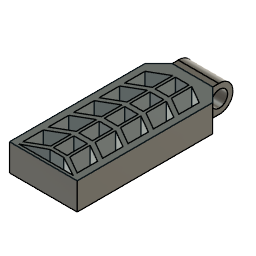
RocketAssembly_GridFin (Autodesk Fusion 360 design; units mm, degrees)
Autodesk Fusion 360 part; units mm, degrees
sketch "Sketch1" plane through (0, 0, 0) normal (0, 0, 1) x (1, 0, 0)
  line L0 (0, 0) -> (12.7, 0)
  line L1 (12.7, 0) -> (12.7, 25.4)
  line L2 (0, 25.4) -> (0, 0)
  line L3 (0, 25.4) -> (2.54, 27.94)
  line L4 (2.54, 27.94) -> (10.16, 27.94)
  line L5 (10.16, 27.94) -> (12.7, 25.4)
  dimension "d1" = 12.7
  dimension "d2" = 25.4
  constraint horizontal L0
  constraint vertical L1
  constraint vertical L2
  constraint coincident L0.start L2.end
  constraint perpendicular L2 L4
  measures "d1" distance of L0.start L0.end
  measures "d2" distance of L0.start L2.start
extrude "Extrude1" add sketch "Sketch1" along normal blind 5.08
sketch "Sketch2" plane through (12.7, 0, 0) normal (1, 0, 0) x (0, 1, 0)
  line L0 (0, 0) -> (25.4, 0)
  line L1 (25.4, 0) -> (25.4, 5.08)
  line L2 (25.4, 5.08) -> (0, 5.08)
  line L3 (0, 5.08) -> (0, 0)
  circle A0 centre (29.21, 2.54) radius 2.54
  circle A1 centre (29.21, 2.54) radius 1.524
  dimension "d5" = 3.048
  constraint concentric A0 A1
  measures "d5" diameter of A1
extrude "Extrude2" add sketch "Sketch2" along normal blind -2.54 and the other way blind 10.16 contours A0
fillet "Fillet1" radius 10.16 1 edges at (6.35, 27.94, 0.3403)
fillet "Fillet2" radius 10.16 1 edges at (6.35, 27.94, 4.7397)
sketch "Sketch3" plane through (0, 0, 5.08) normal (0, 0, 1) x (-1, 0, 0)
  line L0 (0, -25.4) -> (0, 0)
  line L1 (0, 0) -> (-12.7, 0)
  line L2 (-12.7, 0) -> (-12.7, -25.4)
  line L3 (-12.7, -25.4) -> (-10.16, -27.94)
  line L4 (-10.16, -27.94) -> (-2.54, -27.94)
  line L5 (-2.54, -27.94) -> (0, -25.4)
sketch "Sketch4" plane through (0, 0, 0) normal (0, 0, -1) x (1, 0, 0)
  line L0 (0, 0) -> (0, -25.4)
  line L1 (0, -25.4) -> (2.54, -27.94)
  line L2 (2.54, -27.94) -> (10.16, -27.94)
  line L3 (10.16, -27.94) -> (12.7, -25.4)
  line L4 (12.7, -25.4) -> (12.7, 0)
  line L5 (12.7, 0) -> (0, 0)
  line L6 (1.27, -1.27) -> (1.27, -5.08)
  line L7 (1.27, -5.08) -> (4.5696, -6.985)
  line L8 (1.27, -1.27) -> (4.5696, -3.175)
  line L9 (4.5696, -3.175) -> (4.5696, -6.985)
  line L10 (11.43, -1.27) -> (11.43, -5.08)
  line L11 (11.43, -5.08) -> (8.1304, -6.985)
  line L12 (8.1304, -6.985) -> (8.1304, -3.175)
  line L13 (8.1304, -3.175) -> (11.43, -1.27)
  line L14 (1.27, -9.8425) -> (4.5696, -11.7475)
  line L15 (1.27, -6.0325) -> (1.27, -9.8425)
  line L16 (1.27, -6.0325) -> (4.5696, -7.9375)
  line L17 (4.5696, -7.9375) -> (4.5696, -11.7475)
  line L18 (8.1304, -11.7475) -> (8.1304, -7.9375)
  line L19 (8.1304, -7.9375) -> (11.43, -6.0325)
  line L20 (11.43, -6.0325) -> (11.43, -9.8425)
  line L21 (11.43, -9.8425) -> (8.1304, -11.7475)
  line L22 (1.27, -14.605) -> (4.5696, -16.51)
  line L23 (1.27, -10.795) -> (1.27, -14.605)
  line L24 (1.27, -10.795) -> (4.5696, -12.7)
  line L25 (4.5696, -12.7) -> (4.5696, -16.51)
  line L26 (8.1304, -16.51) -> (8.1304, -12.7)
  line L27 (8.1304, -12.7) -> (11.43, -10.795)
  line L28 (11.43, -10.795) -> (11.43, -14.605)
  line L29 (11.43, -14.605) -> (8.1304, -16.51)
  line L30 (1.27, -19.3675) -> (4.5696, -21.2725)
  line L31 (1.27, -15.5575) -> (1.27, -19.3675)
  line L32 (1.27, -15.5575) -> (4.5696, -17.4625)
  line L33 (4.5696, -17.4625) -> (4.5696, -21.2725)
  line L34 (8.1304, -21.2725) -> (8.1304, -17.4625)
  line L35 (8.1304, -17.4625) -> (11.43, -15.5575)
  line L36 (11.43, -15.5575) -> (11.43, -19.3675)
  line L37 (11.43, -19.3675) -> (8.1304, -21.2725)
  line L38 (1.27, -24.13) -> (4.5696, -26.035)
  line L39 (1.27, -20.32) -> (1.27, -24.13)
  line L40 (1.27, -20.32) -> (4.5696, -22.225)
  line L41 (4.5696, -22.225) -> (4.5696, -26.035)
  line L42 (8.1304, -26.035) -> (8.1304, -22.225)
  line L43 (8.1304, -22.225) -> (11.43, -20.32)
  line L44 (11.43, -20.32) -> (11.43, -24.13)
  line L45 (11.43, -24.13) -> (8.1304, -26.035)
  line L46 (5.08, -3.175) -> (7.62, -3.175)
  line L47 (7.62, -3.175) -> (7.62, -6.985)
  line L48 (7.62, -6.985) -> (5.08, -6.985)
  line L49 (5.08, -6.985) -> (5.08, -3.175)
  line L50 (5.08, -3.175) -> (7.62, -6.985) construction
  line L51 (7.62, -3.175) -> (5.08, -6.985) construction
  line L52 (5.08, -7.9375) -> (7.62, -7.9375)
  line L53 (5.08, -11.7475) -> (5.08, -7.9375)
  line L54 (7.62, -11.7475) -> (5.08, -11.7475)
  line L55 (7.62, -7.9375) -> (7.62, -11.7475)
  line L56 (5.08, -12.7) -> (7.62, -12.7)
  line L57 (5.08, -16.51) -> (5.08, -12.7)
  line L58 (7.62, -16.51) -> (5.08, -16.51)
  line L59 (7.62, -12.7) -> (7.62, -16.51)
  line L60 (5.08, -17.4625) -> (7.62, -17.4625)
  line L61 (5.08, -21.2725) -> (5.08, -17.4625)
  line L62 (7.62, -21.2725) -> (5.08, -21.2725)
  line L63 (7.62, -17.4625) -> (7.62, -21.2725)
  line L64 (5.08, -22.225) -> (7.62, -22.225)
  line L65 (5.08, -26.035) -> (5.08, -22.225)
  line L66 (7.62, -26.035) -> (5.08, -26.035)
  line L67 (7.62, -22.225) -> (7.62, -26.035)
  line L68 (5.08, -2.54) -> (7.62, -2.54)
  line L69 (7.62, -2.54) -> (11.43, -0.508)
  line L70 (11.43, -0.508) -> (1.27, -0.508)
  line L71 (1.27, -0.508) -> (5.08, -2.54)
  point P0 (6.35, -5.08)
  dimension "d14" = 120
  dimension "d15" = 3.81
  dimension "d16" = 3.81
  dimension "d17" = 120
  dimension "d18" = 3.81
  dimension "d19" = 3.81
  dimension "d22" = 0
  dimension "d23" = -19.05
  dimension "d24" = 2.54
  dimension "d25" = 3.81
  dimension "d28" = 0
  dimension "d29" = -19.05
  constraint vertical L6
  constraint parallel L7 L8
  constraint parallel L9 L10
  constraint vertical L12
  constraint horizontal L46
  constraint perpendicular L46 L47
  constraint parallel L46 L48
  constraint parallel L47 L49
  constraint coincident L50 P0
  constraint coincident L51 P0
  constraint parallel L5 L68
  constraint parallel L5 L70
  measures "d14" angle of L6 L7
  measures "d15" distance of L6.end L7.end
  measures "d16" distance of L6.start L8.end
  measures "d17" angle of L10 L11
  measures "d18" distance of L10.end L11.end
  measures "d19" distance of L11.end L12.end
  measures "d24" distance of L47.end L48.end
  measures "d25" distance of L46.end L47.end
extrude "Extrude3" cut sketch "Sketch4" against normal blind 7.112 contours L6 L7 L8 L9 | L10 L11 L12 L13 | L14 L15 L16 L17 | L18 L19 L20 L21 | L22 L23 L24 L25 | L26 L27 L28 L29 | L30 L31 L32 L33 | L34 L35 L36 L37 | L38 L39 L40 L41 | L42 L43 L44 L45 | L46 L47 L48 L49 | L52 L53 L54 L55 | L56 L57 L58 L59 | L60 L61 L62 L63 | L64 L65 L66 L67 | L68 L69 L70 L71
